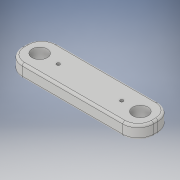
# Autodesk Inventor part: femur_v3
Saved by Autodesk Inventor 2019 (Build 230136000, 136)
## iProperties
Created: 2018-12-28
Part Number: femur_v3
Material: Generic
Document SubType Name: Modeling
Designer: Daniel
Density: 1 g/cm^3
Appearance: Default
Author: Daniel
Autodesk Inventor part; units mm, degrees
ref_plane "YZ Plane" through (0, 0, 0) normal (1, 0, 0) x (0, 1, 0)
ref_plane "XZ Plane" through (0, 0, 0) normal (0, 1, 0) x (-1, 0, 0)
ref_plane "XY Plane" through (0, 0, 0) normal (0, 0, 1) x (1, 0, 0)
sketch "Sketch1" plane through (0, 0, 0) normal (0, 1, 0) x (-1, 0, 0)
  line L0 (42, 0) -> (-42, 0) projected
  line L1 (0, -19.2) -> (0, 3.2) projected
  line L2 (30, -16) -> (-30, -16)
  line L3 (-30, -16) -> (-30, 0)
  line L4 (-30, 0) -> (30, 0)
  line L5 (30, 0) -> (30, -16)
  point P0 (0, 0)
  dimension "d0" = 16
  dimension "d1" = 60
  constraints: 8 end point, 2 parallel, 1 collinear, 1 horizontal, 1 perpendicular, 1 other
  measures "d0" distance between parallel lines of L0 L2
  measures "d1" distance between parallel lines of L3 L5
extrude "Extrusion1" add sketch "Sketch1" along normal blind 6
sketch "Sketch2" plane through (0, 6, 0) normal (0, 1, 0) x (1, 0, 0)
  line L0 (30, 16) -> (-30, 16) projected
  line L1 (-30, 16) -> (-30, 0) projected
  line L2 (-30, 0) -> (30, 0) projected
  line L3 (30, 0) -> (30, 16) projected
  line L4 (0, 19.2) -> (0, -3.2) projected
  line L5 (-42, 0) -> (42, 0) projected
  point P0 (0, 0)
  point P1 (-23, 8)
  point P2 (23, 8)
  dimension "d4" = 7
  dimension "d5" = 7
  dimension "d6" = 8
  dimension "d7" = 8
  measures "d4" distance from line of L1 point (-23, 8)
  measures "d5" distance from line of L3 point (23, 8)
  measures "d6" distance from line of L2 point (23, 8)
  measures "d7" distance from line of L2 point (-23, 8)
hole "Hole1" at (23, 6, -8) at (-23, 6, -8) direction (0, -1, 0) diameter 7 end through all
sketch "Sketch3" plane through (0, 6, 0) normal (0, 1, 0) x (1, 0, 0)
  circle A0 centre (23, 8) radius 3.5 projected
  circle A1 centre (-23, 8) radius 3.5 projected
  line L0 (30, 16) -> (-30, 16) projected
  line L1 (-30, 16) -> (-30, 0) projected
  line L2 (-30, 0) -> (30, 0) projected
  line L3 (30, 0) -> (30, 16) projected
  line L4 (0, 19.2) -> (0, -3.2) projected
  line L5 (-23, 8) -> (23, 8) construction
  point P0 (0, 0)
  point P1 (-14.5, 8)
  point P2 (14.5, 8)
  dimension "d15" = 8.5
  dimension "d16" = 8.5
  constraints: 2 end point, 2 point on line, 1 horizontal
  measures "d15" distance of L5.start point (-14.5, 8)
  measures "d16" distance of L5.end point (14.5, 8)
hole "Hole2" at (-14.5, 6, -8) at (14.5, 6, -8) direction (0, -1, 0) diameter 1.5 end through all
fillet "Fillet1" radius 7 4 edges at (30, 3, -16) (30, 3, 0) (-30, 3, -16) (-30, 3, 0)
fillet "Fillet2" radius 1 16 edges at (0, 0, 0) (-27.9497, 0, -2.0503) (-30, 0, -8) (-27.9497, 0, -13.9497) (0, 0, -16) (27.9497, 0, -13.9497) (30, 0, -8) (27.9497, 0, -2.0503) (27.9497, 6, -2.0503) (30, 6, -8) (27.9497, 6, -13.9497) (0, 6, -16) (-27.9497, 6, -13.9497) (-30, 6, -8) (-27.9497, 6, -2.0503) (0, 6, 0)
body "Solid1"
